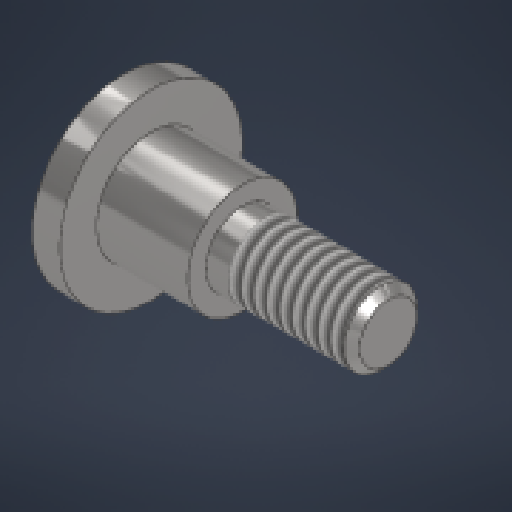
# Autodesk Inventor part: DBGS4-5-8
Saved by Autodesk Inventor 2024.3 (Build 283343000, 343)
## iProperties
Created: 2024-11-01
Part Number: DBGS4-5-8
Material: 스테인리스스틸
Catalog Web Link: www.cadenas.de
Description: DBGB, DBGM, DBGS, DBGSY-Stepped Bolts - Extra Low Head Type
Vendor: MISUMI
Document SubType Name: Modeling
Designer: psAdmin
Manufacturer: MISUMI
Mass: 2.80883 g
Surface Area: 4.09923 cm^2
Volume: 0.351103 cm^3
Density: 8 g/cm^3
Appearance: 반연마
Category: PARTsolutions
Company: MISUMI
PSOL_IDENT_0: {$CADENAS_DATA/23d-libs/misumi/metric/27_screws_nuts/dbgb.prj},198 {VTYP=3D},{NB=DBGS4-5-8},{LINA=DB
PSOL_IDENT_1: GS4-5-8},{NN=DBGB, DBGM, DBGS, DBGSY},{DATE=21.04.2022 12:25:59},{GEOMDATE=18.01.2022 05:16:34},{VER
PSOL_IDENT_2: SION=},{LINEID=20},{WBVAR=MAT,ST,ALT1,L,F,ALT2},{WBNUMERIC=L,F}  {NB=DBGS4-5-8},{LINA=DBGS4-5-8},{KT=
PSOL_IDENT_3: DUMMY},{PN=DBGS4-5-8},{TYPE=DBGS},{MAT=2},{ST=0},{M=4},{ALT1=},{L=5},{F=8},{FA=(3:9/1)},{E=1.5},{D=6
PSOL_IDENT_4: },{A=10},{B=2.0},{LL=1.2},{HH1=2.0},{P=0.70},{ALT2=},{ST0='0','-'},{LINC=[5:20/1]},{GG=0},{FF=0}
NB: DBGS4-5-8
NN: DBGB, DBGM, DBGS, DBGSY
NT: Stepped Bolts - Extra Low Head Type
NBSYN: $PN.
LINA: DBGS4-5-8
CATALOG: Misumi
PN: DBGS4-5-8
MAT: 303 Stainless Steel
ST: -
M: 4
ALT1: w/o LTC (L Dimension Increment)
L: 5
F: 8
E: 1.5
D: 6
A: 10
B: 2
LL: 1.2
HH1: 2
ALT2: w/o PC (Relief on M)
SUPPLIER: MISUMI
ARTICLENO: DBGS4-5-8
BOMINFO: DBGS4-5-8
CREATOR: CADENAS GmbH
Title: DBGS4-5-8
Author: Cadenas PARTsolutions
Comments: Stepped Bolts - Extra Low Head Type
Autodesk Inventor part; units mm, degrees
ref_plane "YZ Plane" through (0, 0, 0) normal (1, 0, 0) x (0, 1, 0)
ref_plane "XZ Plane" through (0, 0, 0) normal (0, 1, 0) x (-1, 0, 0)
ref_plane "XY Plane" through (0, 0, 0) normal (0, 0, 1) x (1, 0, 0)
sketch "Sketch_1" plane through (0, 0, 0) normal (0, 0, 1) x (1, 0, 0)
  line L0 (5, 0) -> (-1.5, 0)
  line L1 (-1.5, 0) -> (-1.5, 5)
  line L2 (-1.5, 5) -> (0, 5)
  line L3 (0, 5) -> (0, 3)
  line L4 (0, 3) -> (5, 3)
  line L5 (5, 3) -> (5, 0)
  line L6 (5, 0) -> (-1.5, 0)
  constraints: 14 end point
revolve "Revolution1" add sketch "Sketch_1" angle 360 about axis through (5, 0, 0) along (1, 0, 0)
sketch "Sketch2" plane through (-1.5, 0, 0) normal (-1, 0, 0) x (0, 0, 1)
  point P0 (0, 0)
hole "Hole1" at (-1.5, 0, 0) direction (1, 0, 0) diameter 2 depth 2 tip angle 120
sketch "Sketch_3" plane through (-1.5, 0, 0) normal (1, 0, 0) x (0, 0, -1)
  line L0 (-1, -0.5774) -> (0, -1.1547)
  line L1 (0, -1.1547) -> (1, -0.5774)
  line L2 (1, -0.5774) -> (1, 0.5774)
  line L3 (1, 0.5774) -> (0, 1.1547)
  line L4 (0, 1.1547) -> (-1, 0.5774)
  line L5 (-1, 0.5774) -> (-1, -0.5774)
  constraints: 12 end point
extrude "Extrusion1" cut sketch "Sketch_3" along normal blind 2
sketch "Sketch_4" plane through (0, 0, 0) normal (0, 0, 1) x (1, 0, 0)
  line L0 (13, 0) -> (5, 0)
  line L1 (5, 0) -> (5, 2)
  line L2 (5, 2) -> (12.5705, 2)
  line L3 (12.5705, 2) -> (13, 1.5705)
  line L4 (13, 1.5705) -> (13, 0)
  line L5 (13, 0) -> (5, 0)
  constraints: 12 end point
revolve "Revolution2" add sketch "Sketch_4" angle 360 about axis through (13, 0, 0) along (1, 0, 0)
thread "Thread1" size "M4x0.7" class "6g" standard "ISO Metric profile" length 6.3705
body "Solid1"
